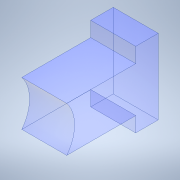
# Autodesk Inventor part: shank_2
Saved by Autodesk Inventor 2020.2 (Build 242310000, 310)
## iProperties
Created: 2021-01-30
Part Number: shank_2
Material: Generic
Document SubType Name: Modeling
Designer: DELL
Density: 1 g/cm^3
Appearance: Clear - Blue
Author: DELL
Autodesk Inventor part; units mm, degrees
ref_plane "YZ Plane" through (0, 0, 0) normal (1, 0, 0) x (0, 1, 0)
ref_plane "XZ Plane" through (0, 0, 0) normal (0, 1, 0) x (-1, 0, 0)
ref_plane "XY Plane" through (0, 0, 0) normal (0, 0, 1) x (1, 0, 0)
sketch "Sketch17" plane through (0, 0, 0) normal (1, 0, 0) x (0, 1, 0)
  line L0 (-67.9, 0) -> (67.9, 0) construction
  line L1 (0, -67.9) -> (0, 67.9) construction
  circle A0 centre (0, 0) radius 40
  circle A1 centre (0, 0) radius 48.5
  dimension "d173" = 97
  dimension "d174" = 80
  constraints: 2 centre point, 2 coincident
  measures "d173" diameter of A1
  measures "d174" diameter of A0
sketch "Sketch16" plane through (0, 0, 0) normal (1, 0, 0) x (0, 1, 0)
  circle A0 centre (0, 0) radius 40
  circle A1 centre (0, 0) radius 48.5
  line L0 (-40, -160) -> (90, -160)
  line L1 (-30, -38.1084) -> (-30, -110) construction
  line L2 (-40, -150) -> (-40, -160) construction
  spline S0 degree 4 poles (-30, -38.1084) (-30, -110) (-40, -110) (-40, -130) (-40, -150) (-40, -160) knots 1 1 1 1 1 1.775953 2 2 2 2 2
  line L3 (30, -38.1084) -> (30, -80) construction
  line L4 (30, -80) -> (30, -90) construction
  line L5 (30, -90) -> (30, -130) construction
  line L6 (30, -130) -> (60, -130) construction
  line L7 (60, -130) -> (90, -130) construction
  line L8 (90, -130) -> (90, -135) construction
  line L9 (90, -135) -> (90, -160) construction
  spline S1 degree 4 poles (30, -38.1084) (30, -80) (30, -90) (30, -130) (60, -130) (90, -130) (90, -135) (90, -160) knots 1 1 1 1 1 2 3 4 5 5 5 5 5
  line L10 (0, -219.1452) -> (0, 93.1075) construction
  line L11 (-30, -110) -> (-40, -110) construction
  line L12 (-40, -110) -> (-40, -130) construction
  line L13 (-40, -130) -> (-40, -150) construction
  dimension "d156" = 97
  dimension "d157" = 80
  dimension "d158" = 160
  dimension "d162" = 60
  dimension "d163" = 30
  dimension "d164" = 90
  dimension "d165" = 5
  dimension "d166" = 40
  dimension "d167" = 80
  dimension "d168" = 10
  dimension "d169" = 10
  dimension "d170" = 20
  dimension "d171" = 40
  dimension "d172" = 20
  constraints: 8 vertical, 4 horizontal, 2 centre point, 2 coincident, 2 end point, 2 point on circle, 1 collinear, 1 perpendicular, 7 other
  measures "d156" diameter of A1
  measures "d157" diameter of A0
  measures "d158" distance from line of L0 point (0, 0)
  measures "d162" distance between parallel lines of L3 L1
  measures "d163" distance from line of L0 L7.end
  measures "d164" distance between parallel lines of L9 L10
  measures "d165" distance of L7.end L8.end
  measures "d166" distance of L5.end L4.end
  measures "d167" distance from line of L0 L3.end
  measures "d168" distance between parallel lines of L1 L12
  measures "d169" distance from line of L0 L2.start
  measures "d170" distance of L2.start L12.end
  measures "d171" distance between parallel lines of L2 L10
  measures "d172" distance of L12.end L11.end
extrude "Extrusion14" add sketch "Sketch16" along normal mid plane 60 contours A1 S1 L0 S0
fillet "Fillet10" radius 5 4 edges at (15, 30, -38.1084) (-15, 30, -38.1084) (15, -30, -38.1084) (-15, -30, -38.1084)
sketch "Sketch18" plane through (0, 0, 0) normal (1, 0, 0) x (0, 1, 0)
  circle A0 centre (0, 0) radius 40 projected
  circle A1 centre (0, 0) radius 48.5 projected
  line L0 (-30, -38.1084) -> (-30, -130)
  line L1 (-30, -130) -> (-50, -130)
  line L2 (-50, -130) -> (-50, -160)
  line L3 (-50, -160) -> (50, -160)
  line L4 (50, -160) -> (50, -130)
  line L5 (50, -130) -> (30, -130)
  line L6 (30, -38.1084) -> (30, -130)
  line L7 (-101.3418, 0) -> (121.8903, 0) construction
  line L8 (0, -238.7311) -> (0, 96.3718) construction
  dimension "d175" = 60
  dimension "d176" = 20
  dimension "d177" = 20
  dimension "d178" = 30
  dimension "d179" = 160
  constraints: 14 end point, 4 perpendicular, 2 point on circle, 2 point on line, 2 vertical, 1 other
  measures "d175" distance between parallel lines of L6 L0
  measures "d176" distance of L0.end L1.end
  measures "d177" distance of L4.end L5.end
  measures "d178" distance of L3.end L4.end
  measures "d179" distance between parallel lines of L3 L7
extrude "Extrusion15" add sketch "Sketch18" along normal mid plane 60 separate body contours A1 L6 L5 L4 L3 L2 L1 L0
body "Solid1"
body "Solid6"
body "Solid7"
